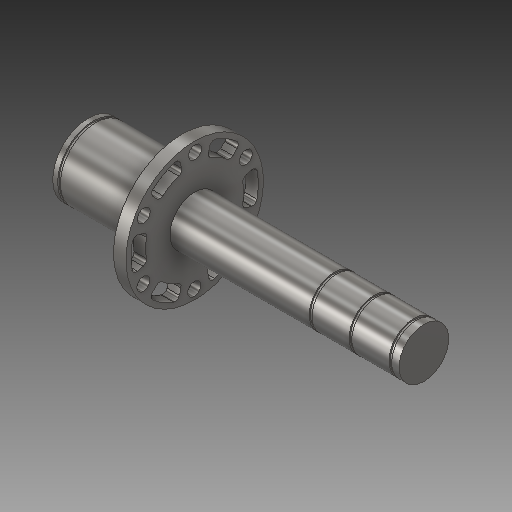
# Autodesk Inventor part: Center Axle
Saved by Autodesk Inventor 2019.4 (Build 234330000, 330)
## iProperties
Created: 2019-12-14
Part Number: Center Axle
Material: Steel, Mild
Document SubType Name: Modeling
Designer: admin
Density: 7.85 g/cm^3
Appearance: Semi-Polished
Author: admin
Autodesk Inventor part; units mm, degrees
ref_plane "YZ Plane" through (0, 0, 0) normal (1, 0, 0) x (0, 1, 0)
ref_plane "XZ Plane" through (0, 0, 0) normal (0, 1, 0) x (-1, 0, 0)
ref_plane "XY Plane" through (0, 0, 0) normal (0, 0, 1) x (1, 0, 0)
sketch "Sketch1" plane through (0, 0, 0) normal (0, 0, 1) x (1, 0, 0)
  line L0 (0, 0) -> (0, 14.3)
  line L1 (115.352, 10) -> (115.352, 9.5)
  line L2 (115.352, 9.5) -> (116.452, 9.5)
  line L3 (116.452, 9.5) -> (116.452, 10)
  line L4 (116.452, 10) -> (131.452, 10)
  line L5 (131.452, 10) -> (131.452, 9.5)
  line L6 (131.452, 9.5) -> (132.552, 9.5)
  line L7 (132.552, 9.5) -> (132.552, 10)
  line L8 (132.552, 10) -> (135.552, 10)
  line L9 (135.552, 10) -> (135.552, 0)
  line L10 (135.552, 0) -> (0, 0)
  line L11 (43, 10) -> (43, 27.75)
  line L12 (43, 27.75) -> (38, 27.75)
  line L13 (0, 14.3) -> (2, 14.3)
  line L14 (2, 14.3) -> (2, 13.8)
  line L15 (2, 13.8) -> (3.1, 13.8)
  line L16 (3.1, 13.8) -> (3.1, 14.3)
  line L17 (3.1, 14.3) -> (38, 14.3)
  line L18 (38, 14.3) -> (38, 27.75)
  line L19 (115.352, 10) -> (100.352, 10)
  line L20 (100.352, 10) -> (100.352, 9.5)
  line L21 (100.352, 9.5) -> (99.252, 9.5)
  line L22 (99.252, 9.5) -> (99.252, 10)
  line L23 (99.252, 10) -> (43, 10)
  dimension "d3" = 1.1
  dimension "d5" = 1.1
  dimension "d6" = 10
  dimension "d8" = 5
  dimension "d9" = 72.352
  dimension "d10" = 27.75
  dimension "d12" = 3
  dimension "d15" = 1.1
  dimension "d16" = 0.5
  dimension "d17" = 2
  dimension "d18" = 34.9
  dimension "d19" = 14.3
  dimension "d20" = 0.5
  dimension "d21" = 0.5
  dimension "d22" = 0.5
  dimension "d23" = 15
  dimension "d39" = 1.1
  dimension "d40" = 0.5
  dimension "d41" = 15
  constraints: 48 end point, 14 perpendicular, 7 point on line, 3 horizontal, 1 vertical
  measures "d3" distance of L1.end L2.end
  measures "d5" distance of L5.end L6.end
  measures "d6" distance between parallel lines of L10 L4
  measures "d8" distance of L11.end L12.end
  measures "d9" distance between parallel lines of L1 L11
  measures "d10" distance between parallel lines of L10 L12
  measures "d12" distance of L7.end L8.end
  measures "d15" distance of L14.end L15.end
  measures "d16" distance of L13.end L14.end
  measures "d17" distance of L0.end L13.end
  measures "d18" distance between parallel lines of L18 L16
  measures "d19" distance between parallel lines of L10 L17
  measures "d20" distance of L1.start L1.end
  measures "d21" distance of L4.end L5.end
  measures "d22" distance of L2.end L3.end
  measures "d23" distance of L3.end L4.end
  measures "d39" distance of L20.end L21.end
  measures "d40" distance of L21.end L22.end
  measures "d41" distance of L1.start L19.end
revolve "Revolution1" add sketch "Sketch1" angle 360 about axis through (135.552, 0, 0) along (-1, 0, 0)
sketch "Sketch2" plane through (43, 0, 0) normal (1, 0, 0) x (0, 0, -1)
  arc A0 (19.9153, -3.9332) -> (19.9669, 3.6623) centre (0, 0) ccw projected
  arc A1 (20.9085, 5.1405) -> (19.9669, 3.6623) centre (21.2333, 3.8946) ccw projected
  line L0 (20.9085, 5.1405) -> (23.1638, 5.7284) projected
  arc A2 (24.7533, 4.7239) -> (23.1638, 5.7284) centre (23.4886, 4.4826) ccw projected
  arc A3 (24.6868, -5.0596) -> (24.7533, 4.7239) centre (0, 0) ccw projected
  arc A4 (23.0839, -6.0425) -> (24.6868, -5.0596) centre (23.4256, -4.8011) ccw projected
  line L1 (23.0839, -6.0425) -> (20.8368, -5.424) construction
  arc A5 (19.9153, -3.9332) -> (20.8368, -5.424) centre (21.1784, -4.1826) ccw projected
  circle A6 centre (20.5409, -12.046) radius 2.1526 construction
  arc A7 (25.2444, 4.8176) -> (23.0377, 6.2122) centre (23.4886, 4.4826) ccw
  line L2 (23.0377, 6.2122) -> (20.7824, 5.6243)
  arc A8 (20.7824, 5.6243) -> (19.4751, 3.5721) centre (21.2333, 3.8946) ccw
  arc A9 (19.4248, -3.8363) -> (19.4751, 3.5721) centre (0, 0) ccw
  arc A10 (19.4248, -3.8363) -> (20.7041, -5.906) centre (21.1784, -4.1826) ccw
  line L3 (20.7041, -5.906) -> (22.9512, -6.5245)
  arc A11 (22.9512, -6.5245) -> (25.1767, -5.16) centre (23.4256, -4.8011) ccw
  arc A12 (25.1767, -5.16) -> (25.2444, 4.8176) centre (0, 0) ccw
  circle A13 centre (20.5409, -12.046) radius 2.6526
  arc A14 (17.126, 16.6141) -> (17.057, 19.2236) centre (15.8707, 17.8866) ccw
  line L4 (15.4668, 14.9772) -> (17.126, 16.6141)
  arc A15 (13.0347, 14.9042) -> (15.4668, 14.9772) centre (14.2115, 16.2497) ccw
  arc A16 (13.0347, 14.9042) -> (6.644, 18.652) centre (0, 0) ccw
  arc A17 (5.5204, 20.8102) -> (6.644, 18.652) centre (7.2438, 20.3359) ccw
  line L5 (6.1389, 23.0574) -> (5.5204, 20.8102)
  arc A18 (8.45, 24.2711) -> (6.1389, 23.0574) centre (7.8623, 22.583) ccw
  arc A19 (17.057, 19.2236) -> (8.45, 24.2711) centre (0, 0) ccw
  circle A20 centre (20.7026, 11.7659) radius 2.6526
  arc A21 (-5.8252, 23.1386) -> (-8.1196, 24.3836) centre (-7.5549, 22.6877) ccw
  line L6 (-5.2373, 20.8833) -> (-5.8252, 23.1386)
  arc A22 (-6.3901, 18.7405) -> (-5.2373, 20.8833) centre (-6.967, 20.4324) ccw
  arc A23 (-6.3901, 18.7405) -> (-12.8311, 15.0799) centre (0, 0) ccw
  arc A24 (-15.262, 15.1859) -> (-12.8311, 15.0799) centre (-13.9895, 16.4412) ccw
  line L7 (-16.8988, 16.8451) -> (-15.262, 15.1859)
  arc A25 (-16.7944, 19.4535) -> (-16.8988, 16.8451) centre (-15.6263, 18.1004) ccw
  arc A26 (-8.1196, 24.3836) -> (-16.7944, 19.4535) centre (0, 0) ccw
  circle A27 centre (0.1617, 23.812) radius 2.6526
  arc A28 (-22.9512, 6.5245) -> (-25.1767, 5.16) centre (-23.4256, 4.8011) ccw
  line L8 (-20.7041, 5.906) -> (-22.9512, 6.5245)
  arc A29 (-19.4248, 3.8363) -> (-20.7041, 5.906) centre (-21.1784, 4.1826) ccw
  arc A30 (-19.4248, 3.8363) -> (-19.4751, -3.5721) centre (0, 0) ccw
  arc A31 (-20.7824, -5.6243) -> (-19.4751, -3.5721) centre (-21.2333, -3.8946) ccw
  line L9 (-23.0377, -6.2122) -> (-20.7824, -5.6243)
  arc A32 (-25.2444, -4.8176) -> (-23.0377, -6.2122) centre (-23.4886, -4.4826) ccw
  arc A33 (-25.1767, 5.16) -> (-25.2444, -4.8176) centre (0, 0) ccw
  circle A34 centre (-20.5409, 12.046) radius 2.6526
  arc A35 (-17.126, -16.6141) -> (-17.057, -19.2236) centre (-15.8707, -17.8866) ccw
  line L10 (-15.4668, -14.9772) -> (-17.126, -16.6141)
  arc A36 (-13.0347, -14.9042) -> (-15.4668, -14.9772) centre (-14.2115, -16.2497) ccw
  arc A37 (-13.0347, -14.9042) -> (-6.644, -18.652) centre (0, 0) ccw
  arc A38 (-5.5204, -20.8102) -> (-6.644, -18.652) centre (-7.2438, -20.3359) ccw
  line L11 (-6.1389, -23.0574) -> (-5.5204, -20.8102)
  arc A39 (-8.45, -24.2711) -> (-6.1389, -23.0574) centre (-7.8623, -22.583) ccw
  arc A40 (-17.057, -19.2236) -> (-8.45, -24.2711) centre (0, 0) ccw
  circle A41 centre (-20.7026, -11.7659) radius 2.6526
  arc A42 (5.8252, -23.1386) -> (8.1196, -24.3836) centre (7.5549, -22.6877) ccw
  line L12 (5.2373, -20.8833) -> (5.8252, -23.1386)
  arc A43 (6.3901, -18.7405) -> (5.2373, -20.8833) centre (6.967, -20.4324) ccw
  arc A44 (6.3901, -18.7405) -> (12.8311, -15.0799) centre (0, 0) ccw
  arc A45 (15.262, -15.1859) -> (12.8311, -15.0799) centre (13.9895, -16.4412) ccw
  line L13 (16.8988, -16.8451) -> (15.262, -15.1859)
  arc A46 (16.7944, -19.4535) -> (16.8988, -16.8451) centre (15.6263, -18.1004) ccw
  arc A47 (8.1196, -24.3836) -> (16.7944, -19.4535) centre (0, 0) ccw
  circle A48 centre (-0.1617, -23.812) radius 2.6526
  point P0 (0, 0)
  dimension "d24" = 0.5
  dimension "d25" = 0.5
  dimension "d28" = 360
  constraints: 72 point on circle, 42 centre point, 24 end point, 152 other
  measures "d24" radial gap between concentric circles of A3 A12
  measures "d25" radial gap between concentric circles of A6 A13
extrude "Extrusion1" cut sketch "Sketch2" against normal through all
sketch "Sketch3" plane through (0, 0, 0) normal (-1, 0, 0) x (0, 0, 1)
  circle A0 centre (0, 0) radius 14.3 projected
  point P0 (0, 0)
  point P1 (0, 0)
  constraints: 1 coincident
hole "Hole1" at (0, 0, 0) direction (1, 0, 0) diameter 15 depth 38
body "Solid1"
